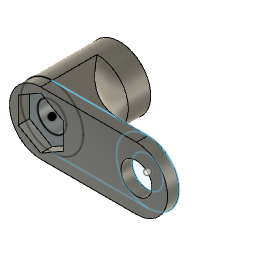
End_Cap_Link_New v1 (Autodesk Fusion 360 design; units mm, degrees)
Autodesk Fusion 360 part; units mm, degrees
sketch "Sketch1" plane through (0, 0, 0) normal (0, 1, 0) x (1, 0, 0)
  circle A0 centre (0, 0) radius 2.55
  circle A1 centre (17, 0) radius 2.75
  circle A2 centre (0, 0) radius 5.55
  circle A3 centre (17, 0) radius 5.55
  line L0 (0.0003, -5.55) -> (17, -5.55)
  line L1 (0.0003, 5.55) -> (17, 5.55)
  dimension "d1" = 5.1
  dimension "d2" = 5.5
  dimension "d3" = 17
  dimension "d4" = 3
  dimension "d5" = 2.8
  constraint coincident A0.centre A2.centre
  constraint coincident A2 L0.start
  constraint coincident A3 L0.end
  constraint tangent A3 L0
  constraint coincident A2 L1.start
  constraint coincident A3 L1.end
  constraint tangent A3 L1
  measures "d1" diameter of A0
  measures "d2" diameter of A1
  measures "d3" distance of A0.centre A1.centre
extrude "Extrude1" add sketch "Sketch1" along normal blind 12 contours A2
extrude "Extrude2" add sketch "Sketch1" against normal blind 2
fillet "Fillet1" radius 8 1 edges at (5.55, 0, 0)
sketch "Sketch2" plane through (0, -2, 0) normal (0, -1, 0) x (1, 0, 0)
  circle A0 centre (0, 0) radius 2.55
  circle A1 centre (17, 0) radius 2.75
  line L0 (0.0003, -5.55) -> (17, -5.55)
  arc A2 (17, -5.55) -> (17, 5.55) centre (17, 0) ccw
  line L1 (17, 5.55) -> (0.0003, 5.55)
  arc A3 (0.0003, 5.55) -> (0.0003, -5.55) centre (0, 0) ccw
  line L2 (4, 2.3094) -> (0, 4.6188)
  line L3 (0, 4.6188) -> (-4, 2.3094)
  line L4 (-4, 2.3094) -> (-4, -2.3094)
  line L5 (-4, -2.3094) -> (0, -4.6188)
  line L6 (0, -4.6188) -> (4, -2.3094)
  line L7 (4, -2.3094) -> (4, 2.3094)
  line L8 (-4.01, -2.3152) -> (0, -4.6303)
  line L9 (0, -4.6303) -> (4.01, -2.3152)
  line L10 (4.01, -2.3152) -> (4.01, 2.3152)
  line L11 (4.01, 2.3152) -> (0, 4.6303)
  line L12 (0, 4.6303) -> (-4.01, 2.3152)
  line L13 (-4.01, 2.3152) -> (-4.01, -2.3152)
  dimension "d12" = 0.01
  constraint coincident A0.centre A3.centre
extrude "Extrude3" cut sketch "Sketch2" against normal blind 2 contours L2 L3 L4 L5 L6 L7 | L8 L9 L10 L11 L12 L13
equation "d1 = 5 mm + 0.1 mm"
equation "d2 = 5 mm + 0.5 mm"
